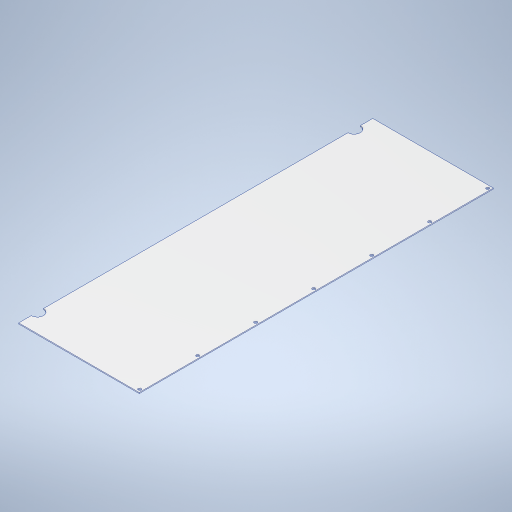
# Autodesk Inventor part: CO-1-01-controlsSeperator
Saved by Autodesk Inventor 2023 (Build 270158000, 158)
## iProperties
Created: 2023-04-06
Part Number: CO-1-01-controlsSeperator
Material: Aluminum 6061
Document SubType Name: Sheet Metal
Designer: t205b
Density: 2.7 g/cm^3
Sheet Metal Rule: Default
Appearance: Aluminum - Flat
Mass: 472.055 g
Surface Area: 2228.99 cm^2
Volume: 174.835 cm^3
Author: t205b
Autodesk Inventor part; units mm, degrees
ref_plane "YZ Plane" through (0, 0, 0) normal (1, 0, 0) x (0, 1, 0)
ref_plane "XZ Plane" through (0, 0, 0) normal (0, 1, 0) x (-1, 0, 0)
ref_plane "XY Plane" through (0, 0, 0) normal (0, 0, 1) x (1, 0, 0)
sketch "Sketch1" plane through (0, 0, 0) normal (0, 1, 0) x (-1, 0, 0)
  line L0 (97, 285) -> (-97, 285)
  line L1 (-97, 285) -> (-97, -285)
  line L2 (-97, -285) -> (97, -285)
  line L3 (97, -285) -> (97, 285)
  point P0 (0, 0)
  dimension "d0" = 194
  dimension "d1" = 570
  dimension "d2" = 97
  dimension "d3" = 285
  measures "d0" distance between parallel lines of L1 L3
  measures "d1" distance of L2.end L0.start
  measures "d2" distance from line of L3 point (0, 0)
  measures "d3" distance from line of point (0, 0) L2
extrude "Plate1" add sketch "Sketch1" along normal blind 1.5875
sketch "Sketch4" plane through (0, 1.5875, 0) normal (0, 1, 0) x (1, 0, 0)
  line L0 (97, -285) -> (-97, -285) projected
  line L1 (97, 285) -> (97, -285) projected
  point P0 (0, 0)
  point P1 (92.8862, -280.075)
  dimension "d22" = 4.925
  dimension "d40" = 4.1138
  measures "d22" distance from line of L0 point (92.886, -280.075)
  measures "d40" distance from line of L1 point (92.886, -280.075)
hole "Hole1" at (92.8862, 1.5875, 280.075) direction (0, -1, 0) diameter 4.9276 end through all
pattern_linear "Rectangular Pattern1" count 7 spacing 93.3583 along (0, 0, -1) of "Hole1"
sketch "Sketch5" plane through (0, 1.5875, 0) normal (0, 1, 0) x (1, 0, 0)
  line L0 (-97, -285) -> (-97, 285) projected
  line L1 (-97, 285) -> (97, 285) projected
  line L2 (97, -285) -> (-97, -285) projected
  point P0 (0, 0)
  point P1 (-97, 255)
  point P2 (-97, -255)
  dimension "d35" = 30
  dimension "d36" = 30
  constraints: 2 point on line
  measures "d35" distance from line of point (-97, 255) L1
  measures "d36" distance from line of L2 point (-97, -255)
hole "Hole2" at (-97, 1.5875, -255) at (-97, 1.5875, 255) direction (0, -1, 0) diameter 20 end through all
equation "\"d20\" = Thickness"
equation "\"d4\" = Thickness"
equation "\"d2\" = 0.5 * d0"
equation "\"d3\" = 0.5 * d1"
equation "\"BendRadius\" = Thickness"
equation "\"BendReliefWidth\" = Thickness"
equation "\"BendReliefDepth\" = 0.5 * Thickness"
equation "\"CornerReliefSize\" = 4 * Thickness"
equation "\"MinimumRemnant\" = 2 * Thickness"
equation "\"TransitionRadius\" = BendRadius"
equation "\"JacobiRadiusSize\" = BendRadius"
equation "\"GapSize\" = Thickness"
equation "\"Thickness\" = 1.5875"
body "Solid1"
